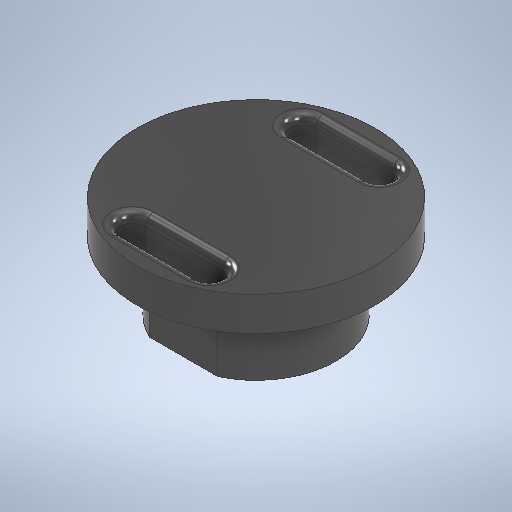
# Autodesk Inventor part: plug
Saved by Autodesk Inventor 2025.2 (Build 292293000, 293)
## iProperties
Created: 2025-04-29
Part Number: plug
Material: Generic
Document SubType Name: Modeling
Designer: 3lin2
Density: 1 g/cm^3
Appearance: Default
Author: 3lin2
Autodesk Inventor part; units mm, degrees
ref_plane "YZ Plane" through (0, 0, 0) normal (1, 0, 0) x (0, 1, 0)
ref_plane "XZ Plane" through (0, 0, 0) normal (0, 1, 0) x (-1, 0, 0)
ref_plane "XY Plane" through (0, 0, 0) normal (0, 0, 1) x (1, 0, 0)
sketch "Sketch1" plane through (0, 0, 0) normal (0, 1, 0) x (-1, 0, 0)
  circle A0 centre (0, 0) radius 11.938
  dimension "d0" = 23.876
  constraints: 1 centre point, 1 coincident
  measures "d0" diameter of A0
extrude "Extrusion1" add sketch "Sketch1" along normal blind 10.16
sketch "Sketch2" plane through (0, 10.16, 0) normal (0, 1, 0) x (1, 0, 0)
  circle A0 centre (0, 0) radius 17.78
  dimension "d3" = 35.56
  constraints: 1 centre point, 1 coincident
  measures "d3" diameter of A0
extrude "Extrusion2" add sketch "Sketch2" along normal blind 5.08
sketch "Sketch3" plane through (0, 15.24, 0) normal (0, 1, 0) x (1, 0, 0)
  line L0 (5.715, -12.7) -> (-5.715, -12.7) construction
  line L1 (5.715, -14.605) -> (-5.715, -14.605)
  line L2 (-5.715, -10.795) -> (5.715, -10.795)
  arc A0 (5.715, -14.605) -> (5.715, -10.795) centre (5.715, -12.7) ccw
  arc A1 (-5.715, -10.795) -> (-5.715, -14.605) centre (-5.715, -12.7) ccw
  line L3 (5.715, 10.795) -> (-5.715, 10.795)
  line L4 (-5.715, 14.605) -> (5.715, 14.605)
  arc A2 (5.715, 10.795) -> (5.715, 14.605) centre (5.715, 12.7) ccw
  arc A3 (-5.715, 14.605) -> (-5.715, 10.795) centre (-5.715, 12.7) ccw
  point P0 (0, 0)
  point P1 (0, -12.7)
  point P2 (7.62, -12.7)
  point P3 (7.62, 12.7)
  point P4 (-7.62, 12.7)
  dimension "d6" = 0
  dimension "d7" = 7.62
  dimension "d8" = 3.81
  dimension "d9" = 3.81
  dimension "d10" = 12.7
  dimension "d11" = 7.62
  dimension "d12" = 7.62
  dimension "d13" = 12.7
  constraints: 12 end point, 11 point on circle, 8 tangent, 4 centre point, 2 parallel, 1 horizontal, 1 midpoint
  measures "d6" horizontal distance of point (0, 0) point (0, -12.7)
  measures "d7" distance of point (7.62, -12.7) point (0, -12.7)
  measures "d8" distance between parallel lines of L2 L1
  measures "d9" distance between parallel lines of L4 L3
  measures "d10" distance of point (0, 0) point (0, -12.7)
  measures "d11" horizontal distance of point (0, 0) point (7.62, 12.7)
  measures "d12" horizontal distance of point (0, 0) point (-7.62, 12.7)
  measures "d13" vertical distance of point (0, 0) A3.centre
extrude "Extrusion3" cut sketch "Sketch3" against normal blind 15.24
fillet "Fillet1" radius 1.27 8 edges at (7.62, 15.24, 12.7) (0, 15.24, 14.605) (-7.62, 15.24, 12.7) (0, 15.24, 10.795) (7.62, 15.24, -12.7) (0, 15.24, -10.795) (-7.62, 15.24, -12.7) (0, 15.24, -14.605)
body "Solid1"
